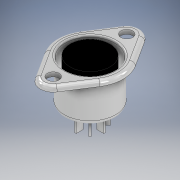
# Autodesk Inventor part: midi_gniazdo
Saved by Autodesk Inventor 2020 (Build 240168000, 168)
## iProperties
Created: 2020-11-28
Part Number: midi_gniazdo
Material: Generic
Document SubType Name: Modeling
Designer: Milosz
Density: 1 g/cm^3
Appearance: Default
Author: Milosz
Autodesk Inventor part; units mm, degrees
ref_plane "YZ Plane" through (0, 0, 0) normal (1, 0, 0) x (0, 1, 0)
ref_plane "XZ Plane" through (0, 0, 0) normal (0, 1, 0) x (-1, 0, 0)
ref_plane "XY Plane" through (0, 0, 0) normal (0, 0, 1) x (1, 0, 0)
sketch "Sketch1" plane through (0, 0, 0) normal (0, 1, 0) x (-1, 0, 0)
  circle A0 centre (0, 0) radius 7.5
  circle A1 centre (0, -10.775) radius 1.725
  circle A2 centre (0, 10.775) radius 1.725
  line L0 (8.1017, 5.1965) -> (3.205, 12.8307)
  line L1 (-3.205, 12.8307) -> (-8.1017, 5.1965)
  line L2 (-8.1017, -5.1965) -> (-3.205, -12.8307)
  line L3 (3.205, -12.8307) -> (8.1017, -5.1965)
  line L4 (0, -20) -> (0, 18) construction
  arc A3 (-3.205, -12.8307) -> (3.205, -12.8307) centre (0, -10.775) ccw
  arc A4 (8.1017, -5.1965) -> (8.1017, 5.1965) centre (0, 0) ccw
  arc A5 (-8.1017, 5.1965) -> (-8.1017, -5.1965) centre (0, 0) ccw
  arc A6 (3.205, 12.8307) -> (-3.205, 12.8307) centre (0, 10.775) ccw
  dimension "d0" = 15
  dimension "d2" = 3.45
  dimension "d4" = 10.775
  dimension "d8" = 3.45
  dimension "d9" = 10.775
  dimension "d34" = 9.625
  dimension "d35" = 9.625
  constraints: 10 end point, 8 point on circle, 8 tangent, 7 centre point, 4 coincident, 3 point on line, 1 vertical
  measures "d0" diameter of A0
  measures "d2" diameter of A2
  measures "d4" distance of A2.centre point (0, 0)
  measures "d8" diameter of A1
  measures "d9" distance of A1.centre point (0, 0)
  measures "d34" radius of A5
  measures "d35" radius of A4
extrude "Extrusion1" add sketch "Sketch1" along normal blind 1.25 contours A0 | A4 L3 A3 L2 A5 L1 A6 L0
fillet "Fillet1" radius 1.25 8 edges at (5.6534, 1.25, 9.0136) (9.625, 1.25, 0) (5.6534, 1.25, -9.0136) (0, 1.25, -14.5826) (-5.6534, 1.25, -9.0136) (-9.625, 1.25, 0) (-5.6534, 1.25, 9.0136) (0, 1.25, 14.5826)
extrude "Extrusion2" add sketch "Sketch1" against normal blind 11.3 contours A0
fillet "Fillet2" radius 1.25 1 edges at (7.5, -11.3, 0)
sketch "Sketch2" plane through (0, -11.3, 0) normal (0, -1, 0) x (1, 0, 0)
  circle A0 centre (0, 0) radius 3.26 construction
  line L0 (-0.25, -2.26) -> (0.25, -2.26)
  line L1 (0.25, -2.26) -> (0.25, -4.26)
  line L2 (0.25, -4.26) -> (-0.25, -4.26)
  line L3 (-0.25, -4.26) -> (-0.25, -2.26)
  line L4 (-0.25, -2.26) -> (0.25, -4.26) construction
  line L5 (0.25, -2.26) -> (-0.25, -4.26) construction
  circle A1 centre (0, 0) radius 3.26 construction
  line L6 (1.4213, -1.7748) -> (1.7748, -1.4213)
  line L7 (1.7748, -1.4213) -> (3.1891, -2.8355)
  line L8 (3.1891, -2.8355) -> (2.8355, -3.1891)
  line L9 (2.8355, -3.1891) -> (1.4213, -1.7748)
  line L10 (1.4213, -1.7748) -> (3.1891, -2.8355) construction
  line L11 (1.7748, -1.4213) -> (2.8355, -3.1891) construction
  circle A2 centre (0, 0) radius 3.26 construction
  line L12 (2.26, -0.25) -> (2.26, 0.25)
  line L13 (2.26, 0.25) -> (4.26, 0.25)
  line L14 (4.26, 0.25) -> (4.26, -0.25)
  line L15 (4.26, -0.25) -> (2.26, -0.25)
  line L16 (2.26, -0.25) -> (4.26, 0.25) construction
  line L17 (2.26, 0.25) -> (4.26, -0.25) construction
  circle A3 centre (0, 0) radius 3.26 construction
  line L18 (1.7748, 1.4213) -> (1.4213, 1.7748)
  line L19 (1.4213, 1.7748) -> (2.8355, 3.1891)
  line L20 (2.8355, 3.1891) -> (3.1891, 2.8355)
  line L21 (3.1891, 2.8355) -> (1.7748, 1.4213)
  line L22 (1.7748, 1.4213) -> (2.8355, 3.1891) construction
  line L23 (1.4213, 1.7748) -> (3.1891, 2.8355) construction
  circle A4 centre (0, 0) radius 3.26 construction
  line L24 (0.25, 2.26) -> (-0.25, 2.26)
  line L25 (-0.25, 2.26) -> (-0.25, 4.26)
  line L26 (-0.25, 4.26) -> (0.25, 4.26)
  line L27 (0.25, 4.26) -> (0.25, 2.26)
  line L28 (0.25, 2.26) -> (-0.25, 4.26) construction
  line L29 (-0.25, 2.26) -> (0.25, 4.26) construction
  point P0 (0, -3.26)
  point P1 (2.3052, -2.3052)
  point P2 (3.26, 0)
  point P3 (2.3052, 2.3052)
  point P4 (0, 3.26)
  dimension "d16" = 6.52
  dimension "d19" = 0.5
  dimension "d20" = 2
  dimension "d23" = 180
  constraints: 60 end point, 10 midpoint, 2 coincident, 2 parallel, 2 vertical alignment, 1 horizontal, 1 horizontal alignment, 1 perpendicular, 64 other
  measures "d19" distance of L1.end L2.end
  measures "d20" distance of L0.end L1.end
extrude "Extrusion3" add sketch "Sketch2" along normal blind 5
sketch "Sketch3" plane through (0, 1.25, 0) normal (0, 1, 0) x (1, 0, 0)
  arc A0 (-7.0495, 4.5216) -> (-7.0495, -4.5216) centre (0, 0) ccw projected
  circle A1 centre (0, 0) radius 7.25
  dimension "d27" = 14.5
  constraints: 1 centre point, 1 coincident
  measures "d27" diameter of A1
extrude "Extrusion4" cut sketch "Sketch3" against normal blind 11.25
sketch "Sketch4" plane through (0, -10, 0) normal (0, 1, 0) x (1, 0, 0)
  circle A0 centre (0, 0) radius 5.85
  dimension "d30" = 11.7
  constraints: 1 centre point, 1 coincident
  measures "d30" diameter of A0
extrude "Extrusion5" add sketch "Sketch4" along normal up to surface (11.25 mm away)
fillet "Fillet3" radius 0.5 1 edges at (-7.25, 1.25, 0)
equation "\"d8\" = d2"
equation "\"d9\" = d4"
equation "\"d35\" = d34"
equation "\"d12\" = d10"
equation "\"d15\" = d10"
equation "\"d10\" = 1.25"
body "Solid1"
